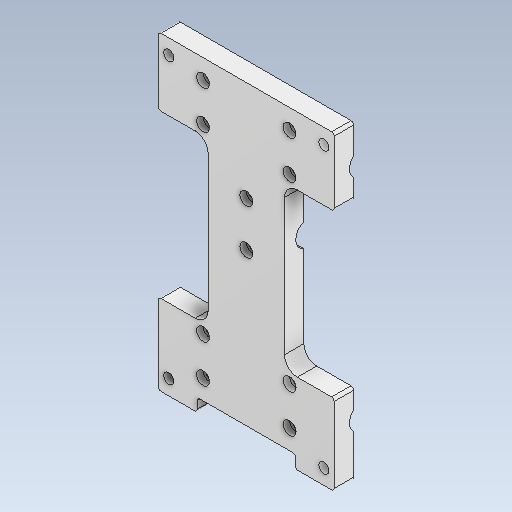
# Autodesk Inventor part: 0008-10-006 suport injectomat
Saved by Autodesk Inventor 2020 (Build 240168000, 168)
## iProperties
Created: 2021-02-26
Part Number: 0008-10-006 suport injectomat
Material: ABS Plastic
Document SubType Name: Modeling
Designer: Iulian Bors
Density: 1.06 g/cm^3
Appearance: Smooth - White
Mass: 330.02 g
Surface Area: 625.949 cm^2
Volume: 311.34 cm^3
Description: Suport Injectomat
Author: Iulian Bors
Subject: 006
Autodesk Inventor part; units mm, degrees
ref_plane "YZ Plane" through (0, 0, 0) normal (1, 0, 0) x (0, 1, 0)
ref_plane "XZ Plane" through (0, 0, 0) normal (0, 1, 0) x (-1, 0, 0)
ref_plane "XY Plane" through (0, 0, 0) normal (0, 0, 1) x (1, 0, 0)
sketch "Sketch1" plane through (0, 0, 0) normal (0, 0, 1) x (1, 0, 0)
  line L0 (-68, 115) -> (68, 115)
  line L1 (68, 115) -> (68, -115)
  line L2 (68, -115) -> (-68, -115)
  line L3 (-68, -115) -> (-68, 115)
  line L4 (-68, -115) -> (-38, -115)
  line L5 (-38, -115) -> (-38, -125)
  line L6 (-38, -125) -> (-68, -125)
  line L7 (-68, -125) -> (-68, -115)
  line L8 (38, -115) -> (68, -115)
  line L9 (68, -115) -> (68, -125)
  line L10 (68, -125) -> (38, -125)
  line L11 (38, -125) -> (38, -115)
  point P0 (0, 0)
  point P1 (0, 115)
  point P2 (-68, 0)
  dimension "d0" = 230
  dimension "d1" = 136
  dimension "d49" = 10
  dimension "d50" = 30
  constraints: 24 end point, 6 parallel, 3 horizontal, 3 perpendicular, 2 collinear, 2 equal length, 2 midpoint, 1 horizontal alignment, 1 vertical alignment
  measures "d0" distance of L2.end L0.start
  measures "d1" distance of L1.end L2.end
  measures "d49" distance of L4.end L5.end
  measures "d50" distance of L5.end L6.end
extrude "Extrusion1" add sketch "Sketch1" along normal blind 15
sketch "Sketch3" plane through (0, 0, 15) normal (0, 0, 1) x (1, 0, 0)
  circle A0 centre (-60, 103.25) radius 4
  circle A1 centre (60, 103.25) radius 4
  circle A2 centre (60, -113.25) radius 4
  circle A3 centre (-60, -113.25) radius 4
  line L0 (68, 115) -> (-68, 115) projected
  line L1 (-68, 115) -> (-68, -125) projected
  line L2 (-38, -115) -> (38, -115) projected
  line L3 (68, -125) -> (68, 115) projected
  point P0 (0, 0)
  point P1 (-68, -115)
  dimension "d10" = 11.75
  dimension "d11" = 8
  dimension "d12" = 8
  dimension "d14" = 1.75
  dimension "d60" = 8
  constraints: 4 centre point, 3 equal radius, 2 horizontal alignment, 2 vertical alignment
  measures "d10" distance from line of A0.centre L0
  measures "d11" diameter of A0
  measures "d12" distance from line of A0.centre L1
  measures "d14" distance from line of L2 A2.centre
  measures "d60" distance from line of A1.centre L3
extrude "Extrusion3" cut sketch "Sketch3" against normal through all
sketch "Sketch2" plane through (68, -115, 0) normal (1, 0, 0) x (0, 0, -1)
  circle A0 centre (6.5, 200) radius 9.75
  circle A1 centre (6.5, 30) radius 9.75
  line L0 (0, 230) -> (-15, 230) projected
  circle A2 centre (3.5, 135) radius 9.75
  line L1 (0, -10) -> (0, 230) projected
  line L2 (0, -10) -> (-15, -10) projected
  point P0 (0, 115)
  dimension "d6" = 19.5
  dimension "d7" = 30
  dimension "d51" = 6.5
  dimension "d53" = 19.5
  dimension "d54" = 40
  dimension "d55" = 20
  dimension "d56" = 3.5
  constraints: 3 centre point, 2 equal radius, 1 vertical alignment
  measures "d6" diameter of A1
  measures "d7" distance from line of A0.centre L0
  measures "d51" distance from line of L1 A0.centre
  measures "d53" diameter of A2
  measures "d54" distance from line of L2 A1.centre
  measures "d55" vertical distance of point (0, 115) A2.centre
  measures "d56" distance from line of L1 A2.centre
extrude "Extrusion2" cut sketch "Sketch2" against normal through all
sketch "Sketch4" plane through (0, 0, 15) normal (0, 0, 1) x (1, 0, 0)
  line L0 (-68, 77.7328) -> (68, 77.7328) projected
  line L1 (68, -77.7328) -> (-68, -77.7328) projected
  circle A0 centre (60, -113.25) radius 4 projected
  circle A1 centre (60, 103.25) radius 4 projected
  circle A2 centre (-60, -113.25) radius 4 projected
  circle A3 centre (-60, 103.25) radius 4 projected
  line L2 (-38, -115) -> (38, -115) projected
  line L3 (68, 115) -> (-68, 115) projected
  line L4 (-14.5, 0) -> (14.5, 0) construction
  line L5 (-68, 62.7328) -> (-29.5, 62.7328)
  line L6 (-29.5, 62.7328) -> (-29.5, -62.7328)
  line L7 (-29.5, -62.7328) -> (-68, -62.7328)
  line L8 (-68, -62.7328) -> (-68, 62.7328)
  line L9 (-68, 115) -> (-68, -125) projected
  line L10 (38, -115) -> (38, -125) projected
  line L11 (38, -125) -> (68, -125) projected
  line L12 (68, -125) -> (68, 115) projected
  line L13 (-68, -125) -> (-38, -125) projected
  line L14 (-38, -125) -> (-38, -115) projected
  line L15 (-68, 115) -> (-68, -125) projected
  point P0 (0, 0)
  point P1 (-68, -115)
  point P2 (0, 0)
  dimension "d18" = 29
  dimension "d19" = 15
  dimension "d20" = 15
  dimension "d21" = 15
  constraints: 10 end point, 2 coincident, 2 horizontal, 2 parallel, 1 collinear, 1 midpoint, 1 perpendicular
  measures "d18" distance of L4.start L4.end
  measures "d19" distance between parallel lines of L5 L0
  measures "d20" distance between parallel lines of L1 L7
  measures "d21" distance from line of L4.start L6
extrude "Extrusion4" cut sketch "Sketch4" against normal through all contours L5 L6 L7 L8
mirror "Mirror1" about plane through (0, 0, 0) normal (1, 0, 0) of "Extrusion4"
sketch "Sketch6" plane through (0, 0, 15) normal (0, 0, 1) x (1, 0, 0)
  circle A0 centre (0, 37.25) radius 2.75
  circle A1 centre (0, 2.75) radius 2.75
  line L0 (-20, -56.5) -> (-20, -71.5) projected
  line L1 (20, -71.5) -> (-20, -71.5) projected
  line L2 (20, -71.5) -> (20, -56.5) projected
  line L3 (20, -56.5) -> (50, -56.5) projected
  line L4 (50, 56.5) -> (50, -56.5) projected
  line L5 (50, 56.5) -> (20, 56.5) projected
  line L6 (20, 56.5) -> (20, 71.5) projected
  line L7 (-20, 71.5) -> (20, 71.5) projected
  line L8 (-20, 71.5) -> (-20, 56.5) projected
  line L9 (-20, 56.5) -> (-50, 56.5) projected
  line L10 (-50, -56.5) -> (-50, 56.5) projected
  line L11 (-50, -56.5) -> (-20, -56.5) projected
  line L12 (29.5, -62.7328) -> (29.5, 62.7328) projected
  line L13 (68, 115) -> (-68, 115) projected
  point P0 (0, 0)
  point P1 (29.5, -52.7328)
  point P2 (29.5, 52.7328)
  point P3 (0, 115)
  dimension "d37" = 5.5
  dimension "d39" = 34.5
  dimension "d40" = 77.75
  constraints: 3 vertical alignment, 1 centre point, 1 midpoint, 2 other
  measures "d37" diameter of A0
  measures "d39" distance of point (0, 2.75) A0.centre
  measures "d40" distance from line of L13 A0.centre
hole "Hole2" at (0, 37.25, 15) at (0, 2.75, 15) direction (0, 0, -1) diameter 5.5 end through all counterbore diameter 10 counterbore depth 5
sketch "Sketch5" plane through (0, 0, 15) normal (0, 0, -1) x (-1, 0, 0)
  circle A0 centre (-60, 103.25) radius 4 projected
  line L0 (-68, -125) -> (-68, 115) projected
  line L1 (-68, 115) -> (68, 115) projected
  point P0 (0, 0)
  point P1 (-33.5, 99.7672)
  point P2 (-33.5, 70.2328)
  point P3 (-68, 62.7328)
  dimension "d57" = 34.5
  dimension "d58" = 15.2328
  dimension "d59" = 29.5344
  constraints: 1 vertical alignment
  measures "d57" distance from line of L0 point (-33.5, 99.767)
  measures "d58" distance from line of point (-33.5, 99.767) L1
  measures "d59" distance of point (-33.5, 99.767) point (-33.5, 70.233)
hole "Hole1" at (33.5, 70.2328, 15) at (33.5, 99.7672, 15) direction (0, 0, -1) diameter 5.5 end through all counterbore diameter 10 counterbore depth 5
mirror "Mirror2" about plane through (0, 0, 0) normal (1, 0, 0) of "Hole1"
mirror "Mirror3" about plane through (0, 0, 0) normal (0, 1, 0) of "Hole1", "Mirror2"
fillet "Fillet2" radius 2 10 edges at (-68, 115, 7.5) (-68, 62.7328, 7.5) (-68, -62.7328, 7.5) (-68, -125, 7.5) (-38, -125, 7.5) (-38, -115, 7.5) (38, -115, 7.5) (38, -125, 7.5) (68, -125, 7.5) (68, 115, 7.5)
fillet "Fillet3" radius 10 4 edges at (-29.5, -62.7328, 7.5) (-29.5, 62.7328, 7.5) (29.5, 62.7328, 7.5) (29.5, -62.7328, 7.5)
sketch "Sketch8" plane through (-66, 62.7328, 0) normal (0, -1, 0) x (1, 0, 0)
  circle A0 centre (1.1275, 4.4625) radius 1.7875 projected
  point P0 (66, 0)
hole "Hole4" at (-64.8725, 62.7328, 4.4625) direction (0, 1, 0) diameter 2.459 depth 8.8 tip angle 118 thread size "M3x0.5" class "6H" standard "ISO Metric profile"
equation "\"d20\" = d19"
equation "\"d21\" = d19"
body "Solid1"
